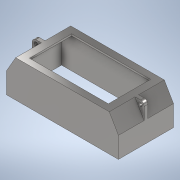
# Autodesk Inventor part: МПСТ Крышка корпуса
Saved by Autodesk Inventor 2022.1 (Build 261234020, 234B)
## iProperties
Created: 2021-11-18
Part Number: МПСТ Крышка корпуса
Material: Сталь, углеродистая
Document SubType Name: Modeling
Designer: Алексанян Г.
Density: 7.85 g/cm^3
Appearance: С умеренной полировкой
Author: Алексанян Г.
Autodesk Inventor part; units mm, degrees
ref_plane "YZ Plane" through (0, 0, 0) normal (1, 0, 0) x (0, 1, 0)
ref_plane "XZ Plane" through (0, 0, 0) normal (0, 1, 0) x (-1, 0, 0)
ref_plane "XY Plane" through (0, 0, 0) normal (0, 0, 1) x (1, 0, 0)
sketch "Эскиз1" plane through (0, 0, 0) normal (0, 1, 0) x (-1, 0, 0)
  line L0 (305, -150) -> (-305, -150)
  line L1 (-305, -150) -> (-305, 150)
  line L2 (-305, 150) -> (305, 150)
  line L3 (305, 150) -> (305, -150)
  line L4 (305, -150) -> (-305, 150) construction
  line L5 (-305, -150) -> (305, 150) construction
  point P0 (0, 0)
  dimension "d0" = 610
  dimension "d1" = 300
  constraints: 12 end point, 2 midpoint, 2 parallel, 1 horizontal, 1 perpendicular
  measures "d0" distance of L1.end L2.end
  measures "d1" distance of L0.end L1.end
extrude "Выдавливание1" add sketch "Эскиз1" along normal blind 200
sketch "Эскиз2" plane through (-305, 0, 150) normal (0, 0, 1) x (1, 0, 0)
  line L0 (0, 200) -> (610, 200) projected
  line L1 (50, 200) -> (0, 113.3975)
  line L2 (0, 0) -> (0, 200) projected
  line L3 (305, -56.4973) -> (305, 277.4189) construction
  line L4 (560, 200) -> (610, 113.3975)
  line L5 (0, 0) -> (610, 0) projected
  line L6 (610, 0) -> (610, 200) projected
  line L7 (610, 113.3975) -> (610, 200)
  point P0 (305, 0)
  point P1 (305, 0)
  dimension "d4" = 60
  dimension "d5" = 50
  constraints: 8 end point, 3 point on line, 2 symmetric about line, 2 vertical, 1 midpoint
  measures "d4" angle of L1 L0
  measures "d5" distance from line of L2 L1.start
extrude "Выдавливание2" cut sketch "Эскиз2" against normal through all contours L0 L1 L2 | L0 L6 L4
sketch "Эскиз3" plane through (0, 0, 0) normal (0, -1, 0) x (1, 0, 0)
  line L0 (-305, 150) -> (305, 150) projected
  point P0 (0, 0)
  point P1 (-228.7398, 140)
  dimension "d8" = 10
  measures "d8" distance from line of L0 point (-228.74, 140)
ref_plane "РабПлоскость1" through (-228.7398, 0, 140) normal (0, 0, 1) x (1, 0, 0)
sketch "Эскиз4" plane through (-228.7398, 0, 140) normal (0, 0, 1) x (1, 0, 0)
  line L0 (483.7398, 200) -> (533.7398, 113.3975) projected
  line L1 (533.7398, 0) -> (533.7398, 113.3975) projected
  line L2 (533.7398, 0) -> (-76.2602, 0) projected
  line L3 (-76.2602, 0) -> (-76.2602, 113.3975) projected
  line L4 (-76.2602, 113.3975) -> (-26.2602, 200) projected
  line L5 (483.7398, 200) -> (-26.2602, 200) projected
  line L6 (-20.4867, 190) -> (-66.2602, 110.718)
  line L7 (-66.2602, 110.718) -> (-66.2602, 0)
  line L8 (523.7398, 0) -> (523.7398, 110.718)
  line L9 (523.7398, 110.718) -> (477.9663, 190)
  line L10 (477.9663, 190) -> (-20.4867, 190)
  line L11 (-66.2602, 0) -> (523.7398, 0)
  line L12 (533.7398, 0) -> (-76.2602, 0) projected
  point P0 (228.7398, 0)
  dimension "d9" = 10
  dimension "d12" = 10
  constraints: 12 end point, 2 point on line, 1 collinear, 3 other
  measures "d9" distance between parallel lines of L5 L10
  measures "d12" distance between parallel lines of L3 L7
extrude "Выдавливание3" cut sketch "Эскиз4" against normal blind 280 contours L2 L7 L6 L10 L9 L8
sketch "Эскиз5" plane through (0, 0, 0) normal (0, 0, 1) x (1, 0, 0)
  line L0 (-255, 200) -> (-305, 200)
  line L1 (-305, 200) -> (-305, 113.3975)
  point P0 (0, 0)
  constraints: 4 end point, 1 horizontal, 1 perpendicular
extrude "Ребро жесткости1" add sketch "Эскиз5" along normal mid plane 20 rib yes fills toward (-280, 199.95) open curves L0 L1
fillet "Сопряжение1" radius 20 1 edges at (-305, 200, 0)
sketch "Эскиз6" plane through (-285, 200, 10) normal (0, 0, 1) x (1, 0, 0)
  arc A0 (0, 0) -> (-20, -20) centre (0, -20) ccw projected
  point P0 (285, -200)
  constraints: 1 coincident
hole "Отверстие1" at (-285, 180, 10) direction (0, 0, -1) diameter 20 end through all
mirror "Зеркальное отражение1" about plane through (0, 0, 0) normal (1, 0, 0) of "Ребро жесткости1", "Отверстие1"
fillet "Сопряжение2" radius 20 1 edges at (305, 200, 0)
sketch "Эскиз7" plane through (0, 200, 0) normal (0, 1, 0) x (1, 0, 0)
  line L0 (215, -115) -> (-215, -115)
  line L1 (-215, -115) -> (-215, 115)
  line L2 (-215, 115) -> (215, 115)
  line L3 (215, 115) -> (215, -115)
  line L4 (215, -115) -> (-215, 115) construction
  line L5 (-215, -115) -> (215, 115) construction
  line L6 (255, 150) -> (-255, 150) projected
  line L7 (-255, 150) -> (-255, 10) projected
  point P0 (0, 0)
  dimension "d28" = 35
  dimension "d29" = 40
  constraints: 12 end point, 2 midpoint, 2 parallel, 1 horizontal, 1 perpendicular
  measures "d28" distance between parallel lines of L2 L6
  measures "d29" distance between parallel lines of L7 L1
extrude "Выдавливание4" cut sketch "Эскиз7" against normal through all
